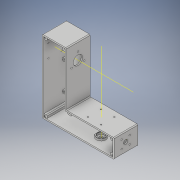
# Autodesk Inventor part: Main Lidar Body
Saved by Autodesk Inventor 2019 (Build 230136000, 136)
## iProperties
Created: 2018-05-20
Part Number: Main Lidar Body
Material: Generic
Document SubType Name: Modeling
Designer: samps
Density: 1 g/cm^3
Appearance: Default
Author: samps
Autodesk Inventor part; units mm, degrees
ref_plane "YZ Plane" through (0, 0, 0) normal (1, 0, 0) x (0, 1, 0)
ref_plane "XZ Plane" through (0, 0, 0) normal (0, 1, 0) x (-1, 0, 0)
ref_plane "XY Plane" through (0, 0, 0) normal (0, 0, 1) x (1, 0, 0)
sketch "Sketch2" plane through (0, 0, 0) normal (0, 0, 1) x (1, 0, 0)
  line L0 (0, 0) -> (0, 3.175)
  line L1 (0, 3.175) -> (50.8, 3.175)
  line L2 (50.8, 3.175) -> (53.975, 3.175)
  line L3 (53.975, 3.175) -> (53.975, -123.825)
  line L4 (53.975, -123.825) -> (108.712, -123.825)
  line L5 (108.712, -123.825) -> (163.449, -123.825)
  line L6 (163.449, -123.825) -> (166.624, -123.825)
  line L7 (166.624, -123.825) -> (166.624, -127)
  line L8 (166.624, -127) -> (166.624, -165.1)
  line L9 (166.624, -165.1) -> (166.624, -168.275)
  line L10 (166.624, -168.275) -> (163.449, -168.275)
  line L11 (163.449, -168.275) -> (0, -168.275)
  line L12 (0, -168.275) -> (-3.175, -168.275)
  line L13 (-3.175, -168.275) -> (-3.175, 0)
  line L14 (-3.175, 0) -> (-3.175, 3.175)
  line L15 (-3.175, 3.175) -> (0, 3.175)
  dimension "d6" = 3.175
  dimension "d13" = 3.175
  dimension "d16" = 3.175
  constraints: 32 end point, 7 point on line, 5 perpendicular, 2 vertical, 1 collinear, 1 horizontal
  measures "d6" distance of L0.start L0.end
  measures "d13" distance of L6.end L7.end
  measures "d16" distance of L9.end L10.end
extrude "Extrusion1" add sketch "Sketch2" along normal blind 55.5625
shell "Shell1" thickness 3.175 removed faces 1 at (15.875, -97.3667, 55.5625)
sketch "Sketch3" plane through (0, -165.1, 3.175) normal (0, 0, 1) x (1, 0, 0)
  line L0 (50.8, 38.1) -> (163.449, 38.1) projected
  line L1 (163.449, 0) -> (0, 0) projected
  line L2 (50.8, 38.1) -> (53.975, 38.1)
  line L3 (53.975, 38.1) -> (53.975, 0)
  line L4 (53.975, 0) -> (50.8, 0)
  line L5 (50.8, 0) -> (50.8, 38.1)
  point P0 (0, 165.1)
  dimension "d21" = 3.175
  constraints: 8 end point, 2 parallel, 1 horizontal, 1 perpendicular, 1 point on line
  measures "d21" distance of L3.end L4.end
extrude "Extrusion2" cut sketch "Sketch3" along normal blind 38.1
sketch "Sketch4" plane through (0, 0, 3.175) normal (0, 0, 1) x (1, 0, 0)
  line L0 (0, 0) -> (50.8, 0) projected
  line L1 (0, 0) -> (6.8, 0)
  line L2 (6.8, 0) -> (6.8, -6.8)
  line L3 (6.8, -6.8) -> (0, -6.8)
  line L4 (0, -6.8) -> (0, 0)
  line L5 (50.8, 0) -> (44, 0)
  line L6 (44, 0) -> (44, -6.8)
  line L7 (44, -6.8) -> (50.8, -6.8)
  line L8 (50.8, -6.8) -> (50.8, 0)
  line L9 (0, -165.1) -> (0, 0) projected
  line L10 (0, -165.1) -> (6.8, -165.1)
  line L11 (6.8, -165.1) -> (6.8, -158.3)
  line L12 (6.8, -158.3) -> (0, -158.3)
  line L13 (0, -158.3) -> (0, -165.1)
  line L14 (50.8, -127) -> (163.449, -127) projected
  line L15 (53.9685, -127) -> (62.7685, -127)
  line L16 (62.7685, -127) -> (62.7685, -133.8)
  line L17 (62.7685, -133.8) -> (53.9685, -133.8)
  line L18 (53.9685, -133.8) -> (53.9685, -127)
  line L19 (163.449, -127) -> (163.449, -165.1) projected
  line L20 (163.449, -127) -> (156.649, -127)
  line L21 (156.649, -127) -> (156.649, -133.8)
  line L22 (156.649, -133.8) -> (163.449, -133.8)
  line L23 (163.449, -133.8) -> (163.449, -127)
  line L24 (163.449, -165.1) -> (156.649, -165.1)
  line L25 (156.649, -165.1) -> (156.649, -158.3)
  line L26 (156.649, -158.3) -> (163.449, -158.3)
  line L27 (163.449, -158.3) -> (163.449, -165.1)
  constraints: 48 end point, 12 parallel, 6 horizontal, 6 perpendicular, 1 point on line
extrude "Extrusion3" add sketch "Sketch4" along normal blind 50.8
sketch "Sketch5" plane through (0, 0, 53.975) normal (0, 0, 1) x (1, 0, 0)
  line L0 (0, -165.1) -> (0, 0) projected
  line L1 (0, 0) -> (2.15, 0)
  line L2 (2.15, 0) -> (2.15, -2.15)
  line L3 (2.15, -2.15) -> (0, -2.15)
  line L4 (0, -2.15) -> (0, 0)
  line L5 (50.8, 0) -> (50.8, -127) projected
  line L6 (50.8, 0) -> (48.65, 0)
  line L7 (48.65, 0) -> (48.65, -2.15)
  line L8 (48.65, -2.15) -> (50.8, -2.15)
  line L9 (50.8, -2.15) -> (50.8, 0)
  line L10 (163.449, -165.1) -> (0, -165.1) projected
  line L11 (0, -165.1) -> (2.15, -165.1)
  line L12 (2.15, -165.1) -> (2.15, -162.95)
  line L13 (2.15, -162.95) -> (0, -162.95)
  line L14 (0, -162.95) -> (0, -165.1)
  line L15 (53.9685, -127) -> (53.9685, -133.8) projected
  line L16 (53.9685, -127) -> (58.3685, -127)
  line L17 (62.7685, -133.8) -> (62.7685, -127) projected
  line L18 (58.3685, -127) -> (58.3685, -129.15)
  line L19 (50.8, -127) -> (163.449, -127) projected
  line L20 (163.449, -127) -> (161.299, -127)
  line L21 (161.299, -127) -> (161.299, -129.15)
  line L22 (161.299, -129.15) -> (163.449, -129.15)
  line L23 (163.449, -129.15) -> (163.449, -127)
  line L24 (163.449, -127) -> (163.449, -165.1) projected
  line L25 (163.449, -165.1) -> (161.299, -165.1)
  line L26 (161.299, -165.1) -> (161.299, -162.95)
  line L27 (161.299, -162.95) -> (163.449, -162.95)
  line L28 (163.449, -162.95) -> (163.449, -165.1)
  constraints: 44 end point, 10 parallel, 7 perpendicular, 5 horizontal, 1 point on line
hole "Hole1" at (2.15, -2.15, 53.975) at (48.65, -2.15, 53.975) at (2.15, -162.95, 53.975) at (58.3685, -129.15, 53.975) at (161.299, -129.15, 53.975) at (161.299, -162.95, 53.975) direction (0, 0, -1) diameter 3.5 depth 3.5
fillet "Fillet1" radius 2 5 edges at (53.975, 3.175, 27.7812) (166.624, -123.825, 27.7812) (166.624, -168.275, 27.7812) (-3.175, -168.275, 27.7812) (-3.175, 3.175, 27.7812)
fillet "Fillet2" radius 2 7 edges at (6.8, -158.3, 28.575) (6.8, -6.8, 28.575) (44, -6.8, 28.575) (62.7685, -133.8, 28.575) (53.9685, -133.8, 28.575) (156.649, -158.3, 28.575) (156.649, -133.8, 28.575)
sketch "Sketch6" plane through (53.975, -123.825, 55.5625) normal (1, 0, 0) x (0, 0, -1)
  line L0 (52.3875, 123.825) -> (1.5875, 123.825) projected
  line L1 (52.3875, 123.825) -> (52.3875, 88.825)
  line L2 (52.3875, -34.475) -> (52.3875, 117.025) projected
  line L3 (52.3875, 88.825) -> (26.9875, 88.825)
  line L4 (0, 123.825) -> (0, -3.175) projected
  point P0 (55.5625, 123.825)
  dimension "d58" = 35
  dimension "d59" = 25.4
  constraints: 4 end point, 1 perpendicular, 1 point on line
  measures "d58" distance of L0.start L1.end
  measures "d59" distance of L1.end L3.end
hole "Hole2" at (53.975, -35, 28.575) direction (-1, 0, 0) diameter 22 depth 3.175
sketch "Sketch7" plane through (53.975, -123.825, 55.5625) normal (0, 1, 0) x (1, 0, 0)
  line L0 (0, 52.3875) -> (0, 14.2875) projected
  line L1 (0, 52.3875) -> (54.737, 52.3875)
  line L2 (102.674, 52.3875) -> (-47.175, 52.3875) projected
  line L3 (54.737, 52.3875) -> (54.737, 26.9875)
  point P0 (-53.975, 55.5625)
  dimension "d67" = 54.737
  dimension "d68" = 25.4
  constraints: 4 end point, 1 perpendicular, 1 point on line
  measures "d67" distance of L0.start L1.end
  measures "d68" distance of L1.end L3.end
hole "Hole3" at (108.712, -123.825, 28.575) direction (0, -1, 0) diameter 15.5 end through all
sketch "Sketch8" plane through (53.975, -123.825, 55.5625) normal (1, 0, 0) x (0, 0, -1)
  circle A0 centre (26.9875, 88.825) radius 11 projected
  line L0 (26.9875, 88.825) -> (26.9875, 106.275)
  line L1 (26.9875, 88.825) -> (42.0996, 80.1)
  line L2 (26.9875, 88.825) -> (44.4375, 88.825) construction
  line L3 (26.9875, 88.825) -> (11.8754, 80.1)
  line L4 (26.9875, 88.825) -> (44.4375, 88.825) construction
  point P0 (55.5625, 123.825)
  dimension "d76" = 17.45
  dimension "d77" = 17.45
  dimension "d78" = 30
  dimension "d79" = 17.45
  dimension "d80" = 150
  constraints: 10 end point, 2 equal length, 2 horizontal, 1 vertical
  measures "d76" distance of L0.start L0.end
  measures "d77" distance of L0.start L1.end
  measures "d78" angle of L1 L2
  measures "d79" distance of L0.start L3.end
  measures "d80" angle of L3 L4
hole "Hole4" at (53.975, -17.55, 28.575) at (53.975, -43.725, 13.4629) at (53.975, -43.725, 43.6871) direction (-1, 0, 0) diameter 3.5 depth 3.175
sketch "Sketch9" plane through (-3.175, -166.275, 0) normal (-1, 0, 0) x (0, 0, 1)
  circle A0 centre (28.575, 131.275) radius 11 projected
  line L0 (28.575, 146.775) -> (13.075, 146.775)
  line L1 (13.075, 146.775) -> (44.075, 146.775)
  line L2 (44.075, 146.775) -> (44.075, 115.775)
  line L3 (44.075, 115.775) -> (13.075, 115.775)
  line L4 (13.075, 115.775) -> (13.075, 146.775)
  point P0 (0, 166.275)
  dimension "d90" = 31
  dimension "d91" = 31
  constraints: 10 end point, 2 parallel, 1 coincident, 1 horizontal, 1 perpendicular
  measures "d90" distance of L2.end L3.end
  measures "d91" distance of L1.end L2.end
hole "Hole5" at (-3.175, -50.5, 13.075) at (-3.175, -19.5, 13.075) at (-3.175, -19.5, 44.075) at (-3.175, -50.5, 44.075) direction (1, 0, 0) diameter 3 depth 3.175
sketch "Sketch10" plane through (50.8, -127, 55.5625) normal (-1, 0, 0) x (0, 0, 1)
  line L0 (-14.2875, -38.1) -> (-52.3875, -38.1) projected
  line L1 (-52.3875, -38.1) -> (-38.2875, -38.1)
  line L2 (-38.2875, -38.1) -> (-38.2875, -24)
  line L3 (-38.2875, -24) -> (-38.2875, -12.5)
  line L4 (-38.2875, -12.5) -> (-49.7875, -12.5)
  line L5 (-49.7875, -12.5) -> (-26.7875, -12.5)
  line L6 (-26.7875, -12.5) -> (-26.7875, -35.5)
  line L7 (-26.7875, -35.5) -> (-49.7875, -35.5)
  line L8 (-49.7875, -35.5) -> (-49.7875, -12.5)
  point P0 (-55.5625, 127)
  dimension "d99" = 14.1
  dimension "d100" = 14.1
  dimension "d101" = 11.5
  dimension "d102" = 11.5
  dimension "d103" = 23
  dimension "d104" = 23
  constraints: 16 end point, 2 horizontal, 2 parallel, 2 perpendicular, 2 point on line
  measures "d99" distance of L0.end L1.end
  measures "d100" distance of L1.end L2.end
  measures "d101" distance of L2.end L3.end
  measures "d102" distance of L3.end L4.end
  measures "d103" distance of L6.end L7.end
  measures "d104" distance of L5.end L6.end
hole "Hole6" at (50.8, -139.5, 5.775) at (50.8, -139.5, 28.775) at (50.8, -162.5, 28.775) at (50.8, -162.5, 5.775) direction (1, 0, 0) diameter 2.5 depth 3.175
sketch "Sketch11" plane through (166.624, -166.275, 0) normal (1, 0, 0) x (0, 0, -1)
  line L0 (-53.975, 39.275) -> (-53.975, 34.475) projected
  line L1 (-53.975, 39.275) -> (-49.575, 39.275)
  line L2 (-3.175, 39.275) -> (-53.975, 39.275) projected
  line L3 (-49.575, 39.275) -> (-49.575, 37.125)
  line L4 (-50.475, 38.875) -> (-50.475, 35.375) projected
  line L5 (-3.175, 34.475) -> (-3.175, 39.275) projected
  line L6 (-3.175, 39.275) -> (-7.575, 39.275)
  line L7 (-7.575, 39.275) -> (-7.575, 37.125)
  line L8 (-53.975, 1.175) -> (-3.175, 1.175) projected
  line L9 (-53.975, 1.175) -> (-49.575, 1.175)
  line L10 (-49.575, 1.175) -> (-49.575, 3.325)
  line L11 (-3.175, 1.175) -> (-3.175, 5.975) projected
  line L12 (-3.175, 1.175) -> (-7.575, 1.175)
  line L13 (-7.575, 1.175) -> (-7.575, 3.325)
  point P0 (0, 166.275)
  dimension "d112" = 4.4
  dimension "d113" = 2.15
  dimension "d114" = 90
  dimension "d115" = 4.4
  dimension "d116" = 2.15
  dimension "d117" = 4.4
  dimension "d118" = 2.15
  dimension "d119" = 4.4
  dimension "d120" = 2.15
  constraints: 16 end point, 4 point on line, 3 perpendicular, 1 parallel
  measures "d112" distance of L0.start L1.end
  measures "d113" distance of L1.end L3.end
  measures "d114" angle of L1 L3
  measures "d115" distance of L2.start L6.end
  measures "d116" distance of L6.end L7.end
  measures "d117" distance of L8.start L9.end
  measures "d118" distance of L9.end L10.end
  measures "d119" distance of L8.end L12.end
  measures "d120" distance of L12.end L13.end
hole "Hole7" at (166.624, -129.15, 49.575) at (166.624, -129.15, 7.575) at (166.624, -162.95, 49.575) at (166.624, -162.95, 7.575) direction (-1, 0, 0) diameter 3.5 depth 3.175
fillet "Fillet3" radius 2 2 edges at (50.8, -127, 29.3688) (53.975, -123.825, 27.7812)
sketch "Sketch12" plane through (0, -165.1, 41.275) normal (0, 0, 1) x (1, 0, 0)
  point P0 (0, 165.1)
sketch "Sketch13" plane through (6.8, -165.1, 3.175) normal (0, 0, 1) x (1, 0, 0)
  line L0 (47.1685, 38.1) -> (47.1685, 33.3) projected
  line L1 (149.849, 0) -> (0, 0) projected
  line L2 (47.1685, 38.1) -> (55.9685, 38.1) projected
  line L3 (44, 158.3) -> (44, 40.1) projected
  line L4 (44, 0) -> (35.2, 0)
  line L5 (35.2, 0) -> (35.2, 6.8)
  line L6 (35.2, 6.8) -> (44, 6.8)
  line L7 (44, 0) -> (44, 6.8)
  point P0 (-6.8, 165.1)
  dimension "d137" = 8.8
  dimension "d138" = 6.8
  constraints: 8 end point, 2 perpendicular, 2 point on line
  measures "d137" distance of L4.start L4.end
  measures "d138" distance of L4.end L5.end
extrude "Extrusion4" add sketch "Sketch13" along normal blind 50.8
sketch "Sketch14" plane through (6.8, -165.1, 53.975) normal (0, 0, 1) x (1, 0, 0)
  line L0 (44, 6.8) -> (35.2, 6.8) projected
  line L1 (44, 6.8) -> (39.6, 6.8)
  line L2 (35.2, 6.8) -> (35.2, 0) projected
  line L3 (39.6, 6.8) -> (39.6, 3.4)
  point P0 (-6.8, 165.1)
  dimension "d141" = 4.4
  constraints: 4 end point, 2 perpendicular
  measures "d141" distance of L0.start L1.end
hole "Hole8" at (46.4, -161.7, 53.975) direction (0, 0, -1) diameter 3.5 depth 3.5
sketch "Sketch15" plane through (0, 0, 53.975) normal (0, 0, 1) x (1, 0, 0)
  line L0 (52.8, -127) -> (53.9685, -127) projected
  line L1 (53.9685, -127) -> (62.7685, -127)
  line L2 (62.7685, -127) -> (62.7685, -133.8)
  line L3 (62.7685, -133.8) -> (53.9685, -133.8)
  line L4 (53.9685, -133.8) -> (53.9685, -127)
  line L5 (50.8, -158.3) -> (42, -158.3) projected
  line L6 (50.8, -165.1) -> (42, -165.1) projected
  line L7 (50.8, -158.3) -> (42, -158.3)
  line L8 (42, -158.3) -> (42, -165.1)
  line L9 (42, -165.1) -> (50.8, -165.1)
  line L10 (50.8, -165.1) -> (50.8, -158.3)
  point P0 (0, 0)
  constraints: 16 end point, 4 parallel, 2 horizontal, 2 perpendicular
fillet "Fillet4" radius 2 2 edges at (42, -158.3, 28.575) (50.8, -158.3, 28.575)
extrude "Extrusion5" cut sketch "Sketch15" against normal blind 1.5875
sketch "Sketch16" plane through (0, 0, 52.3875) normal (0, 0, 1) x (1, 0, 0)
  circle A0 centre (58.3685, -129.15) radius 1.75 projected
  circle A1 centre (46.4, -161.7) radius 1.75 projected
  point P0 (0, 0)
  constraints: 2 coincident
hole "Hole9" at (58.3685, -129.15, 52.3875) at (46.4, -161.7, 52.3875) direction (0, 0, -1) diameter 3.5 depth 3.5
sketch "Sketch17" plane through (0, 0, 52.3875) normal (0, 0, 1) x (1, 0, 0)
  line L0 (42, -165.1) -> (6.8, -165.1) projected
  line L1 (42, -165.1) -> (50.8, -165.1)
  line L2 (50.8, -165.1) -> (50.8, -158.3)
  line L3 (50.8, -158.3) -> (42, -158.3)
  line L4 (42, -158.3) -> (42, -165.1)
  point P0 (0, 0)
  constraints: 8 end point, 2 parallel, 1 horizontal, 1 perpendicular
extrude "Extrusion6" cut sketch "Sketch17" against normal blind 49.2125
sketch "Sketch18" plane through (6.8, -165.1, 3.175) normal (0, 0, 1) x (1, 0, 0)
  line L0 (44, 158.3) -> (44, 40.1) projected
  line L1 (44, 40.1) -> (44, 0)
  line L2 (156.649, 0) -> (-6.8, 0) projected
  line L3 (44, 0) -> (44, 6)
  line L4 (44, 6) -> (40.6, 6)
  line L5 (40.6, 6) -> (40.6, 10.4)
  point P0 (-6.8, 165.1)
  dimension "d161" = 6
  dimension "d162" = 3.4
  dimension "d163" = 4.4
  constraints: 8 end point, 2 perpendicular, 2 point on line, 1 vertical
  measures "d161" distance of L1.end L3.end
  measures "d162" distance of L3.end L4.end
  measures "d163" distance of L4.end L5.end
hole "Hole10" at (47.4, -154.7, 3.175) direction (0, 0, -1) diameter 3.5 depth 3.5
delete faces "Delete1" heal yes whole lump no faces at (109.3356, -124.8833, 36.2999) (109.9552, -166.1583, 36.2246)
sketch "Sketch19" plane through (-1.175, -168.275, 0) normal (0, -1, 0) x (1, 0, 0)
  point P0 (1.175, 0)
  point P1 (109.887, 28.575)
  point P2 (109.887, 28.575)
  constraints: 1 coincident
hole "Hole11" at (108.712, -168.275, 28.575) direction (0, 1, 0) diameter 7.5 depth 3.175
sketch "Sketch20" plane through (0, -165.1, 55.5625) normal (0, 1, 0) x (1, 0, 0)
  circle A0 centre (108.712, 26.9875) radius 3.75 projected
  circle A1 centre (108.712, 26.9875) radius 8
  circle A2 centre (108.712, 26.9875) radius 11
  point P0 (0, 55.5625)
  dimension "d178" = 16
  dimension "d179" = 22
  constraints: 2 centre point, 2 coincident
  measures "d178" diameter of A1
  measures "d179" diameter of A2
extrude "Extrusion7" add sketch "Sketch20" along normal blind 5 contours A2
fillet "Fillet5" radius 0.5 1 edges at (100.712, -160.1, 28.575)
fillet "Fillet6" radius 0.5 1 edges at (97.712, -160.1, 28.575)
sketch "Sketch21" plane through (52.8, -127, 55.5625) normal (0, -1, 0) x (1, 0, 0)
  point P0 (-52.8, -55.5625)
sketch "Sketch22" plane through (6.8, 0, 3.175) normal (0, 0, 1) x (1, 0, 0)
  line L0 (55.9685, -127) -> (55.9685, -131.8) projected
  line L1 (46, -127) -> (156.649, -127) projected
  line L2 (90.912, -165.1) -> (90.912, -160.6) projected
  line L3 (90.912, -165.1) -> (112.912, -165.1) projected
  line L4 (156.649, -165.1) -> (-6.8, -165.1) projected
  point P0 (-6.8, 0)
  constraints: 1 point on line
delete faces "Delete2" heal yes whole lump no faces at (165.5657, -130.5056, 6.4682) (165.5657, -128.0987, 48.176) (165.5657, -161.6879, 50.7873) (165.5657, -164.3056, 6.4682)
sketch "Sketch23" plane through (166.624, -166.275, 0) normal (1, 0, 0) x (0, 0, -1)
  line L0 (-3.175, 34.475) -> (-3.175, 39.275) projected
  line L1 (-53.975, 1.575) -> (-53.975, 5.075) projected
  line L2 (-3.175, 39.275) -> (-53.975, 39.275)
  line L3 (-53.975, 39.275) -> (-53.975, 1.575)
  line L4 (-53.975, 1.575) -> (-3.175, 1.575)
  line L5 (-3.175, 1.575) -> (-3.175, 39.275)
  line L6 (-53.975, 39.275) -> (-28.575, 39.275)
  line L7 (-3.175, 39.275) -> (-53.975, 39.275) projected
  line L8 (-28.575, 39.275) -> (-28.575, 20.425)
  line L9 (-39.575, 1.175) -> (-17.575, 1.175) projected
  line L10 (-28.575, 20.425) -> (-28.575, 29.925)
  line L11 (-28.575, 29.925) -> (-19.075, 29.925)
  line L12 (-19.075, 29.925) -> (-38.075, 29.925)
  line L13 (-38.075, 29.925) -> (-38.075, 10.925)
  line L14 (-38.075, 10.925) -> (-19.075, 10.925)
  line L15 (-19.075, 10.925) -> (-19.075, 29.925)
  point P0 (0, 166.275)
  dimension "d187" = 9.5
  dimension "d188" = 9.5
  dimension "d189" = 19
  dimension "d190" = 19
  constraints: 24 end point, 4 parallel, 4 perpendicular, 2 horizontal, 1 midpoint, 1 point on line
  measures "d187" distance of L8.end L10.end
  measures "d188" distance of L10.end L11.end
  measures "d189" distance of L14.end L13.end
  measures "d190" distance of L13.end L12.end
hole "Hole12" at (166.624, -136.35, 38.075) at (166.624, -136.35, 19.075) at (166.624, -155.35, 19.075) at (166.624, -155.35, 38.075) direction (-1, 0, 0) diameter 3.5 depth 3.5
sketch "Sketch24" plane through (166.624, -166.275, 0) normal (1, 0, 0) x (0, 0, -1)
  circle A0 centre (-38.075, 29.925) radius 1.75 projected
  circle A1 centre (-19.075, 29.925) radius 1.75 projected
  line L0 (-38.075, 29.925) -> (-19.075, 29.925)
  line L1 (-19.075, 29.925) -> (-28.575, 29.925)
  line L2 (-28.575, 29.925) -> (-28.575, 20.425)
  point P0 (0, 166.275)
  dimension "d198" = 9.5
  constraints: 6 end point, 1 horizontal, 1 midpoint, 1 vertical
  measures "d198" distance of L1.end L2.end
hole "Hole13" at (166.624, -145.85, 28.575) direction (-1, 0, 0) diameter 10 depth 3.5
sketch "Sketch25" plane through (108.712, -160.1, 28.575) normal (0, 1, 0) x (1, 0, 0)
  circle A0 centre (0, 0) radius 11 projected
  line L0 (0, 0) -> (-11, 0)
  line L1 (-11, 0) -> (-11, 11)
  line L2 (-11, 11) -> (-11, -11)
  line L3 (-11, -11) -> (-9, -11)
  line L4 (-9, -11) -> (-9, 11)
  line L5 (-9, 11) -> (-11, 11)
  point P0 (-108.712, 28.575)
  dimension "d206" = 11
  dimension "d207" = 22
  dimension "d208" = 2
  constraints: 12 end point, 2 perpendicular, 1 horizontal, 1 horizontal alignment, 1 parallel, 1 point on line, 1 vertical, 1 other
  measures "d206" distance of L0.end L1.end
  measures "d207" distance of L1.end L2.end
  measures "d208" distance of L2.end L3.end
extrude "Extrusion8" cut sketch "Sketch25" against normal blind 5 contours L4 L0 A0 | A0 L1 L5 L4 | L4 L3 L2 A0 | A0 L0 L4
sketch "Sketch26" plane through (55.975, -123.825, 0) normal (0, 1, 0) x (1, 0, 0)
  circle A0 centre (52.737, -28.575) radius 8 projected
  line L0 (52.737, -28.575) -> (68.237, -28.575)
  line L1 (68.237, -28.575) -> (68.237, -13.075)
  line L2 (68.237, -13.075) -> (37.237, -13.075)
  line L3 (37.237, -13.075) -> (37.237, -44.075)
  line L4 (37.237, -44.075) -> (68.237, -44.075)
  line L5 (68.237, -44.075) -> (68.237, -13.075)
  point P0 (-55.975, 0)
  dimension "d211" = 15.5
  dimension "d212" = 15.5
  dimension "d213" = 31
  dimension "d214" = 31
  constraints: 12 end point, 2 horizontal, 2 parallel, 2 perpendicular, 1 coincident
  measures "d211" distance of L0.start L0.end
  measures "d212" distance of L0.end L1.end
  measures "d213" distance of L4.end L3.end
  measures "d214" distance of L3.end L2.end
hole "Hole14" at (93.212, -123.825, 13.075) at (93.212, -123.825, 44.075) at (124.212, -123.825, 44.075) at (124.212, -123.825, 13.075) direction (0, -1, 0) diameter 3 depth 3.5
sketch "Sketch27" plane through (6.8, 0, 3.175) normal (0, 0, 1) x (1, 0, 0)
  line L0 (-6.8, -158.3) -> (-6.8, -6.8) projected
  line L1 (-6.8, -35.0971) -> (-6.8, -56.3471)
  line L2 (-6.8, -56.3471) -> (-6.8, -61.3471)
  line L3 (-6.8, -61.3471) -> (-6.8, -131.3471)
  arc A0 (44, -125) -> (46, -127) centre (46, -125) ccw projected
  line L4 (46, -127) -> (46, -165.3359)
  line L5 (46, -165.3359) -> (46, -127)
  line L6 (44, -6.8) -> (44, -125) projected
  line L7 (44, -125) -> (44, -165.3359)
  line L8 (46, -146.168) -> (44, -146.168)
  line L9 (44, -35.0971) -> (44, -146.168)
  line L10 (44, -146.168) -> (44, -90.6325)
  line L11 (44, -90.6325) -> (44, -55.6325)
  line L12 (-6.8, -55.6325) -> (-6.8, -125.6325)
  line L13 (44, -125.6325) -> (44, -55.6325)
  line L14 (-6.8, -55.6325) -> (-4.4, -55.6325)
  line L15 (-6.8, -61.3471) -> (-6.8, -66.8471)
  line L16 (44, 0) -> (44, -125) projected
  line L17 (44, -66.8471) -> (44, -136.8471)
  line L18 (-6.8, -136.8471) -> (-6.8, -66.8471)
  line L19 (-6.8, -66.8471) -> (-4.4, -66.8471)
  line L20 (44, -66.8471) -> (41.6, -66.8471)
  line L21 (-6.8, -136.8471) -> (-4.4, -136.8471)
  line L22 (44, -136.8471) -> (41.6, -136.8471)
  line L23 (44, -146.168) -> (41.6, -146.168)
  line L24 (-6.8, -146.168) -> (-4.4, -146.168)
  line L25 (-4.4, -136.8471) -> (-4.4, -134.8471)
  line L26 (-4.4, -66.8471) -> (-4.4, -68.8471)
  line L27 (41.6, -66.8471) -> (41.6, -68.8471)
  line L28 (41.6, -136.8471) -> (41.6, -134.8471)
  line L29 (-4.4, -146.168) -> (-4.4, -144.168)
  line L30 (41.6, -146.168) -> (41.6, -144.168)
  circle A1 centre (-4.4, -68.8471) radius 3.75
  circle A2 centre (41.6, -68.8471) radius 3.75
  circle A3 centre (-4.4, -134.8471) radius 3.75
  circle A4 centre (41.6, -134.8471) radius 3.75
  point P0 (-6.8, 0)
  dimension "d222" = 21.25
  dimension "d223" = 5
  dimension "d229" = 5.5
  dimension "d230" = 70
  dimension "d231" = 2.4
  dimension "d232" = 2
  dimension "d233" = 2
  dimension "d234" = 2
  dimension "d235" = 7.5
  dimension "d236" = 7.5
  dimension "d237" = 7.5
  dimension "d238" = 7.5
  constraints: 56 end point, 12 point on line, 8 vertical, 4 centre point, 4 coincident, 2 collinear, 2 midpoint, 2 parallel, 1 perpendicular
  measures "d222" distance of L1.start L1.end
  measures "d223" distance of L1.end L2.end
  measures "d229" distance of L2.end L15.end
  measures "d230" distance of L17.start L17.end
  measures "d231" distance of L17.start L20.end
  measures "d232" distance of L21.end L25.end
  measures "d233" distance of L19.end L26.end
  measures "d234" distance of L24.end L29.end
  measures "d235" diameter of A1
  measures "d236" diameter of A2
  measures "d237" diameter of A3
  measures "d238" diameter of A4
extrude "Extrusion9" add sketch "Sketch27" along normal blind 7.5 contours A3 L0 | L0 A3 | A1 L0 | L0 A1 | A4 L7 | L7 A4 | A2 L6 | L6 A2
sketch "Sketch28" plane through (6.8, 0, 10.675) normal (0, 0, 1) x (1, 0, 0)
  arc A0 (-6.8, -71.7285) -> (-6.8, -65.9657) centre (-4.4, -68.8471) ccw projected
  arc A1 (44, -65.9657) -> (44, -71.7285) centre (41.6, -68.8471) ccw projected
  circle A2 centre (41.6, -134.8471) radius 3.75 projected
  arc A3 (-6.8, -137.7285) -> (-6.8, -131.9657) centre (-4.4, -134.8471) ccw projected
  point P0 (-6.8, 0)
  constraints: 4 coincident
hole "Hole15" at (2.4, -68.8471, 10.675) at (48.4, -68.8471, 10.675) at (48.4, -134.8471, 10.675) at (2.4, -134.8471, 10.675) direction (0, 0, -1) diameter 3.5 depth 3.5
body "Solid1"
